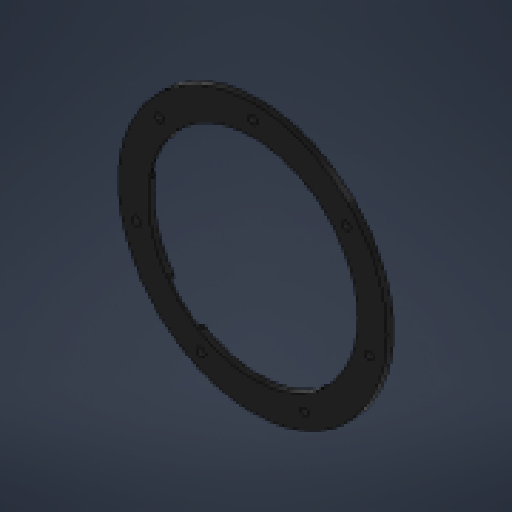
# Autodesk Inventor part: 3DPRINT,TURRET,SPACER
Saved by Autodesk Inventor 2026.1 (Build 301233020, 233B)
## iProperties
Created: 2026-02-09
Part Number: 3DPRINT,TURRET,SPACER
Material: Nylon 6/6
Document SubType Name: Modeling
Designer: littl
Density: 1.13 g/cm^3
Appearance: Smooth - Black
Author: littl
Autodesk Inventor part; units mm, degrees
ref_plane "YZ Plane" through (0, 0, 0) normal (1, 0, 0) x (0, 1, 0)
ref_plane "XZ Plane" through (0, 0, 0) normal (0, 1, 0) x (-1, 0, 0)
ref_plane "XY Plane" through (0, 0, 0) normal (0, 0, 1) x (1, 0, 0)
sketch "Sketch1" plane through (0, 0, 0) normal (0, 0, 1) x (1, 0, 0)
  circle A0 centre (0, 0) radius 79.375
  circle A1 centre (0, 0) radius 101.6
  dimension "d0" = 158.75
  dimension "d1" = 203.2
  constraints: 2 centre point, 2 coincident
  measures "d0" diameter of A0
  measures "d1" diameter of A1
extrude "Extrusion1" add sketch "Sketch1" along normal blind 4.826
sketch "Sketch2" plane through (0, 0, 4.826) normal (0, 0, 1) x (1, 0, 0)
  point P0 (0, 0)
  point P1 (0, 90.4875)
  point P2 (-70.746, 56.418)
  point P3 (-88.2188, -20.1354)
  point P4 (-39.2611, -81.5264)
  point P5 (39.2611, -81.5264)
  point P6 (88.2188, -20.1354)
  point P7 (70.746, 56.418)
  dimension "d4" = 90.4875
  dimension "d7" = 360
  constraints: 1 vertical alignment, 8 other
  measures "d4" distance of point (0, 0) point (0, 90.487)
hole "Hole1" at (0, 90.4875, 4.826) at (-70.746, 56.418, 4.826) at (-88.2188, -20.1354, 4.826) at (-39.2611, -81.5264, 4.826) at (39.2611, -81.5264, 4.826) at (88.2188, -20.1354, 4.826) at (70.746, 56.418, 4.826) direction (0, 0, -1) diameter 6.35 end through all
sketch "Sketch3" plane through (0, 0, 0) normal (0, 0, -1) x (-1, 0, 0)
  arc A0 (90.3392, 17.794) -> (78.8052, 47.6188) centre (0, 0) ccw
  line L0 (0, 0) -> (90.3392, 17.794)
  line L1 (0, 0) -> (78.8052, 47.6188)
  arc A1 (50.34, -77.0953) -> (73.6723, -55.2286) centre (0, 0) ccw
  line L2 (0, 0) -> (50.34, -77.0953)
  line L3 (0, 0) -> (73.6723, -55.2286)
  circle A2 centre (88.2188, -20.1354) radius 3.175 projected
  line L4 (88.2188, -20.1354) -> (0, 0)
  circle A3 centre (0, 0) radius 79.375 construction
  arc A4 (77.8787, 15.3397) -> (67.9355, 41.0507) centre (0, 0) ccw
  arc A5 (43.3966, -66.4615) -> (63.5106, -47.6109) centre (0, 0) ccw
  dimension "d16" = 92.075
  dimension "d17" = 20
  dimension "d18" = 20
  dimension "d19" = 24
  constraints: 13 point on circle, 10 end point, 5 coincident, 4 centre point, 4 point on line, 1 symmetric about line
  measures "d16" radius of A0
  measures "d17" angle of L0 L1
  measures "d18" angle of L2 L3
  measures "d19" angle of L0 L4
extrude "Extrusion2" cut sketch "Sketch3" against normal blind 3.175 contours L0 A4 L1 A0 | A5 L3 A1 L2
fillet "Fillet1" radius 3.175 8 edges at (-78.8052, 47.6188, 1.5875) (-90.3392, 17.794, 1.5875) (-77.8787, 15.3397, 1.5875) (-67.9355, 41.0507, 1.5875) (-73.6723, -55.2286, 1.5875) (-63.5106, -47.6109, 1.5875) (-43.3966, -66.4615, 1.5875) (-50.34, -77.0953, 1.5875)
body "Solid1"
